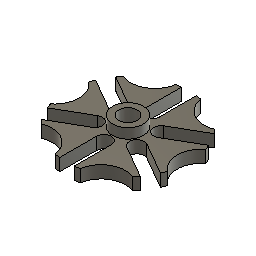
Geneva_wheel (Autodesk Fusion 360 design; units mm, degrees)
Autodesk Fusion 360 part; units mm, degrees
sketch "Sketch1" plane through (0, 0, 0) normal (0, 1, 0) x (1, 0, 0)
  line L0 (6, 19.6387) -> (6, 49.6387)
  line L1 (-6, 19.6387) -> (-6, 49.6387)
  arc A0 (-6, 19.6387) -> (6, 19.6387) centre (0, 19.6387) ccw
  line L2 (-20.0076, 4.6232) -> (-45.9884, 19.6232)
  arc A1 (-20.0076, 4.6232) -> (-14.0076, 15.0155) centre (-17.0076, 9.8193) ccw
  line L3 (-14.0076, 15.0155) -> (-39.9884, 30.0155)
  line L4 (-14.0076, -15.0155) -> (-39.9884, -30.0155)
  arc A2 (-14.0076, -15.0155) -> (-20.0076, -4.6232) centre (-17.0076, -9.8193) ccw
  line L5 (-20.0076, -4.6232) -> (-45.9884, -19.6232)
  line L6 (6, -19.6387) -> (6, -49.6387)
  arc A3 (6, -19.6387) -> (-6, -19.6387) centre (0, -19.6387) ccw
  line L7 (-6, -19.6387) -> (-6, -49.6387)
  line L8 (20.0076, -4.6232) -> (45.9884, -19.6232)
  arc A4 (20.0076, -4.6232) -> (14.0076, -15.0155) centre (17.0076, -9.8193) ccw
  line L9 (14.0076, -15.0155) -> (39.9884, -30.0155)
  line L10 (14.0076, 15.0155) -> (39.9884, 30.0155)
  arc A5 (14.0076, 15.0155) -> (20.0076, 4.6232) centre (17.0076, 9.8193) ccw
  line L11 (20.0076, 4.6232) -> (45.9884, 19.6232)
  arc A6 (47.5, 15.6125) -> (47.5, -15.6125) centre (60, 0) ccw
  arc A7 (45.9884, -19.6232) -> (47.5, -15.6125) centre (0, 0) ccw
  arc A8 (47.5, 15.6125) -> (45.9884, 19.6232) centre (0, 0) ccw
  arc A9 (10.2292, 48.9425) -> (37.2708, 33.33) centre (30, 51.9615) ccw
  arc A10 (-37.2708, 33.33) -> (-10.2292, 48.9425) centre (-30, 51.9615) ccw
  arc A11 (-47.5, -15.6125) -> (-47.5, 15.6125) centre (-60, 0) ccw
  arc A12 (-10.2292, -48.9425) -> (-37.2708, -33.33) centre (-30, -51.9615) ccw
  arc A13 (37.2708, -33.33) -> (10.2292, -48.9425) centre (30, -51.9615) ccw
  arc A14 (39.9884, 30.0155) -> (37.2708, 33.33) centre (0, 0) ccw
  arc A15 (10.2292, 48.9425) -> (6, 49.6387) centre (0, 0) ccw
  arc A16 (-6, 49.6387) -> (-10.2292, 48.9425) centre (0, 0) ccw
  arc A17 (-37.2708, 33.33) -> (-39.9884, 30.0155) centre (0, 0) ccw
  arc A18 (-45.9884, 19.6232) -> (-47.5, 15.6125) centre (0, 0) ccw
  arc A19 (-47.5, -15.6125) -> (-45.9884, -19.6232) centre (0, 0) ccw
  arc A20 (-39.9884, -30.0155) -> (-37.2708, -33.33) centre (0, 0) ccw
  arc A21 (-10.2292, -48.9425) -> (-6, -49.6387) centre (0, 0) ccw
  arc A22 (6, -49.6387) -> (10.2292, -48.9425) centre (0, 0) ccw
  arc A23 (37.2708, -33.33) -> (39.9884, -30.0155) centre (0, 0) ccw
  dimension "d1" = 100
  dimension "d2" = 12
  dimension "d3" = 30
  dimension "d5" = 360
  dimension "d6" = 40
  dimension "d7" = 60
  dimension "d9" = 360
  constraint coincident A7.centre A8.centre
  constraint tangent L0 A0
  constraint tangent L1 A0
  constraint vertical L1
  constraint parallel L0 L1
  constraint vertical A7.centre A0.centre
  constraint concentric A16 A18
  constraint concentric A18 A20
  constraint concentric A20 A22
  constraint concentric A7 A22
  constraint concentric A7 A14
  constraint coincident A6.start A7
  constraint concentric A7 A8
  constraint concentric A14 A15
  constraint concentric A16 A17
  constraint concentric A18 A19
  constraint concentric A20 A21
  constraint concentric A22 A23
  measures "d1" diameter of A16
  measures "d2" diameter of A0
  measures "d3" distance of L0.start L0.end
  measures "d6" diameter of A6
  measures "d7" distance of A7.centre A6.centre
extrude "Extrude1" add sketch "Sketch1" along normal blind 10
sketch "Sketch2" plane through (0, 0, 0) normal (0, -1, 0) x (1, 0, 0)
  line L0 (6, 49.6387) -> (6, 19.6387)
  arc A0 (-6, 19.6387) -> (6, 19.6387) centre (0, 19.6387) ccw
  line L1 (-6, 19.6387) -> (-6, 49.6387)
  arc A1 (-6, 49.6387) -> (-10.2292, 48.9425) centre (0, 0) ccw
  arc A2 (-37.2708, 33.33) -> (-10.2292, 48.9425) centre (-30, 51.9615) ccw
  arc A3 (-37.2708, 33.33) -> (-39.9884, 30.0155) centre (0, 0) ccw
  line L2 (-39.9884, 30.0155) -> (-14.0076, 15.0155)
  arc A4 (-20.0076, 4.6232) -> (-14.0076, 15.0155) centre (-17.0076, 9.8193) ccw
  line L3 (-20.0076, 4.6232) -> (-45.9884, 19.6232)
  arc A5 (-45.9884, 19.6232) -> (-47.5, 15.6125) centre (0, 0) ccw
  arc A6 (-47.5, -15.6125) -> (-47.5, 15.6125) centre (-60, 0) ccw
  arc A7 (-47.5, -15.6125) -> (-45.9884, -19.6232) centre (0, 0) ccw
  line L4 (-45.9884, -19.6232) -> (-20.0076, -4.6232)
  arc A8 (-14.0076, -15.0155) -> (-20.0076, -4.6232) centre (-17.0076, -9.8193) ccw
  line L5 (-14.0076, -15.0155) -> (-39.9884, -30.0155)
  arc A9 (-39.9884, -30.0155) -> (-37.2708, -33.33) centre (0, 0) ccw
  arc A10 (-10.2292, -48.9425) -> (-37.2708, -33.33) centre (-30, -51.9615) ccw
  arc A11 (-10.2292, -48.9425) -> (-6, -49.6387) centre (0, 0) ccw
  line L6 (-6, -49.6387) -> (-6, -19.6387)
  arc A12 (6, -19.6387) -> (-6, -19.6387) centre (0, -19.6387) ccw
  line L7 (6, -19.6387) -> (6, -49.6387)
  arc A13 (6, -49.6387) -> (10.2292, -48.9425) centre (0, 0) ccw
  arc A14 (37.2708, -33.33) -> (10.2292, -48.9425) centre (30, -51.9615) ccw
  arc A15 (37.2708, -33.33) -> (39.9884, -30.0155) centre (0, 0) ccw
  line L8 (39.9884, -30.0155) -> (14.0076, -15.0155)
  arc A16 (20.0076, -4.6232) -> (14.0076, -15.0155) centre (17.0076, -9.8193) ccw
  line L9 (20.0076, -4.6232) -> (45.9884, -19.6232)
  arc A17 (45.9884, -19.6232) -> (47.5, -15.6125) centre (0, 0) ccw
  arc A18 (47.5, 15.6125) -> (47.5, -15.6125) centre (60, 0) ccw
  arc A19 (47.5, 15.6125) -> (45.9884, 19.6232) centre (0, 0) ccw
  line L10 (45.9884, 19.6232) -> (20.0076, 4.6232)
  arc A20 (14.0076, 15.0155) -> (20.0076, 4.6232) centre (17.0076, 9.8193) ccw
  line L11 (14.0076, 15.0155) -> (39.9884, 30.0155)
  arc A21 (39.9884, 30.0155) -> (37.2708, 33.33) centre (0, 0) ccw
  arc A22 (10.2292, 48.9425) -> (37.2708, 33.33) centre (30, 51.9615) ccw
  arc A23 (10.2292, 48.9425) -> (6, 49.6387) centre (0, 0) ccw
  circle A24 centre (0, 0) radius 12.5
  dimension "d12" = 25
  constraint concentric A1 A24
  measures "d12" diameter of A24
extrude "Extrude2" add sketch "Sketch2" along normal blind 8 contours A24
sketch "Sketch3" plane through (0, 10, 0) normal (0, 1, 0) x (-1, 0, 0)
  line L0 (-6, 19.6387) -> (-6, 49.6387)
  arc A0 (-6, 49.6387) -> (-10.2292, 48.9425) centre (0, 0) ccw
  arc A1 (-37.2708, 33.33) -> (-10.2292, 48.9425) centre (-30, 51.9615) ccw
  arc A2 (-37.2708, 33.33) -> (-39.9884, 30.0155) centre (0, 0) ccw
  line L1 (-39.9884, 30.0155) -> (-14.0076, 15.0155)
  arc A3 (-20.0076, 4.6232) -> (-14.0076, 15.0155) centre (-17.0076, 9.8193) ccw
  line L2 (-20.0076, 4.6232) -> (-45.9884, 19.6232)
  arc A4 (-45.9884, 19.6232) -> (-47.5, 15.6125) centre (0, 0) ccw
  arc A5 (-47.5, -15.6125) -> (-47.5, 15.6125) centre (-60, 0) ccw
  arc A6 (-47.5, -15.6125) -> (-45.9884, -19.6232) centre (0, 0) ccw
  line L3 (-45.9884, -19.6232) -> (-20.0076, -4.6232)
  arc A7 (-14.0076, -15.0155) -> (-20.0076, -4.6232) centre (-17.0076, -9.8193) ccw
  line L4 (-14.0076, -15.0155) -> (-39.9884, -30.0155)
  arc A8 (-39.9884, -30.0155) -> (-37.2708, -33.33) centre (0, 0) ccw
  arc A9 (-10.2292, -48.9425) -> (-37.2708, -33.33) centre (-30, -51.9615) ccw
  arc A10 (-10.2292, -48.9425) -> (-6, -49.6387) centre (0, 0) ccw
  line L5 (-6, -49.6387) -> (-6, -19.6387)
  arc A11 (6, -19.6387) -> (-6, -19.6387) centre (0, -19.6387) ccw
  line L6 (6, -19.6387) -> (6, -49.6387)
  arc A12 (6, -49.6387) -> (10.2292, -48.9425) centre (0, 0) ccw
  arc A13 (37.2708, -33.33) -> (10.2292, -48.9425) centre (30, -51.9615) ccw
  arc A14 (37.2708, -33.33) -> (39.9884, -30.0155) centre (0, 0) ccw
  line L7 (39.9884, -30.0155) -> (14.0076, -15.0155)
  arc A15 (20.0076, -4.6232) -> (14.0076, -15.0155) centre (17.0076, -9.8193) ccw
  line L8 (20.0076, -4.6232) -> (45.9884, -19.6232)
  arc A16 (45.9884, -19.6232) -> (47.5, -15.6125) centre (0, 0) ccw
  arc A17 (47.5, 15.6125) -> (47.5, -15.6125) centre (60, 0) ccw
  arc A18 (47.5, 15.6125) -> (45.9884, 19.6232) centre (0, 0) ccw
  line L9 (45.9884, 19.6232) -> (20.0076, 4.6232)
  arc A19 (14.0076, 15.0155) -> (20.0076, 4.6232) centre (17.0076, 9.8193) ccw
  line L10 (14.0076, 15.0155) -> (39.9884, 30.0155)
  arc A20 (39.9884, 30.0155) -> (37.2708, 33.33) centre (0, 0) ccw
  arc A21 (10.2292, 48.9425) -> (37.2708, 33.33) centre (30, 51.9615) ccw
  arc A22 (10.2292, 48.9425) -> (6, 49.6387) centre (0, 0) ccw
  line L11 (6, 49.6387) -> (6, 19.6387)
  arc A23 (-6, 19.6387) -> (6, 19.6387) centre (0, 19.6387) ccw
  circle A24 centre (0, 0) radius 7.5
  dimension "d15" = 15
  constraint concentric A0 A24
  measures "d15" diameter of A24
extrude "Extrude3" cut sketch "Sketch3" against normal blind 30 contours A24
move_body "Move1" bodies 1 to x (1, 0, 0) y (0, -1, 0) z (0, 0, -1) at (0, -16, -99.2774)
